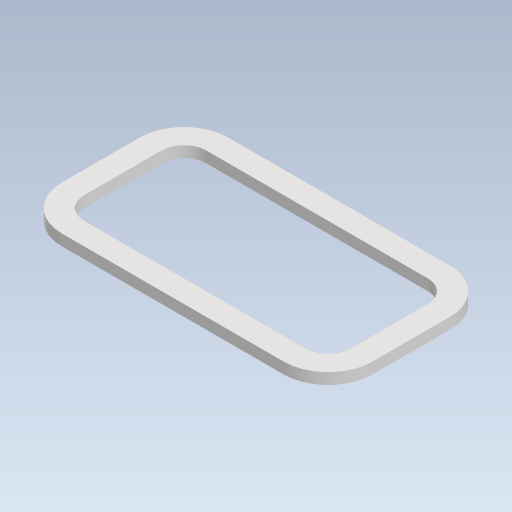
# Autodesk Inventor part: base-plate
Saved by Autodesk Inventor 2023 (Build 270158030, 158C)
## iProperties
Created: 2024-12-17
Part Number: base-plate
Material: Generic
Document SubType Name: Modeling
Designer: Imogen Heard
Density: 1 g/cm^3
Appearance: Default
Author: Imogen Heard
Autodesk Inventor part; units mm, degrees
ref_plane "YZ Plane" through (0, 0, 0) normal (1, 0, 0) x (0, 1, 0)
ref_plane "XZ Plane" through (0, 0, 0) normal (0, 1, 0) x (-1, 0, 0)
ref_plane "XY Plane" through (0, 0, 0) normal (0, 0, 1) x (1, 0, 0)
sketch "Sketch1" plane through (0, 0, 0) normal (0, 1, 0) x (-1, 0, 0)
  line L0 (-20, -75) -> (-120, -75)
  line L1 (-140, -55) -> (-140, -20)
  line L2 (-120, 0) -> (-20, 0)
  line L3 (0, -20) -> (0, -55)
  line L4 (-120, -65) -> (-20, -65)
  line L5 (-10, -55) -> (-10, -20)
  line L6 (-20, -10) -> (-120, -10)
  line L7 (-130, -20) -> (-130, -55)
  arc A0 (-20, -65) -> (-10, -55) centre (-20, -55) ccw
  arc A1 (-10, -20) -> (-20, -10) centre (-20, -20) ccw
  arc A2 (-120, -10) -> (-130, -20) centre (-120, -20) ccw
  arc A3 (-130, -55) -> (-120, -65) centre (-120, -55) ccw
  arc A4 (-20, -75) -> (0, -55) centre (-20, -55) ccw
  arc A5 (-140, -55) -> (-120, -75) centre (-120, -55) ccw
  arc A6 (-120, 0) -> (-140, -20) centre (-120, -20) ccw
  arc A7 (0, -20) -> (-20, 0) centre (-20, -20) ccw
  point P0 (0, 0)
  point P1 (0, 0)
  dimension "d0" = 75
  dimension "d1" = 140
  dimension "d2" = 10
  dimension "d3" = 10
  dimension "d4" = 20
  constraints: 16 end point, 16 point on circle, 16 tangent, 8 centre point, 6 equal radius, 4 parallel, 2 perpendicular, 2 point on line, 1 coincident, 1 horizontal, 3 other
  measures "d0" distance between parallel lines of L2 L0
  measures "d1" distance between parallel lines of L1 L3
  measures "d2" distance between parallel lines of L4 L0
  measures "d3" radius of A0
  measures "d4" radius of A4
extrude "Extrusion1" add sketch "Sketch1" along normal blind 5
body "Solid1"
